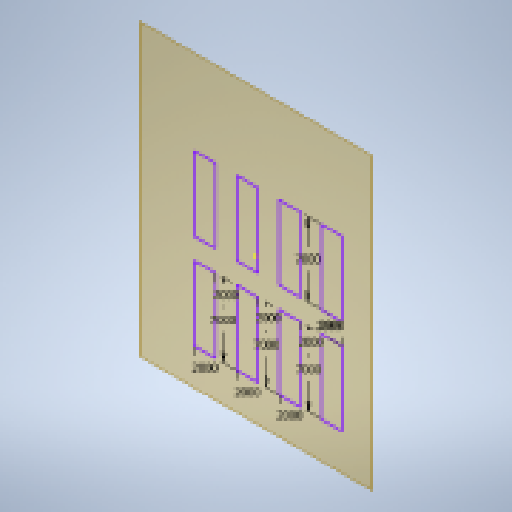
# Autodesk Inventor part: farm pot
Saved by Autodesk Inventor 2025 (Build 290162010, 162A)
## iProperties
Created: 2024-06-18
Part Number: farm pot
Material: 일반
Document SubType Name: Modeling
Designer: user
Density: 1 g/cm^3
Appearance: 기본값
Author: user
Autodesk Inventor part; units mm, degrees
ref_plane "YZ Plane" through (0, 0, 0) normal (1, 0, 0) x (0, 1, 0)
ref_plane "XZ Plane" through (0, 0, 0) normal (0, 1, 0) x (-1, 0, 0)
ref_plane "XY Plane" through (0, 0, 0) normal (0, 0, 1) x (1, 0, 0)
ref_plane "작업 평면1" through (0, 0, 0) normal (0, 0, 1) x (1, 0, 0)
ref_plane "작업 평면2" through (0, 0, 0) normal (0, 0, 1) x (1, 0, 0)
sketch "스케치1" plane through (0, 0, 0) normal (0, 0, 1) x (1, 0, 0)
  line L0 (8181.2099, -11309.2966) -> (6181.2099, -11309.2966)
  line L1 (6181.2099, -11309.2966) -> (6181.2099, -4309.2966)
  line L2 (6181.2099, -4309.2966) -> (8181.2099, -4309.2966)
  line L3 (8181.2099, -4309.2966) -> (8181.2099, -11309.2966)
  line L4 (4181.2099, -4309.2966) -> (2181.2099, -4309.2966)
  line L5 (2181.2099, -4309.2966) -> (2181.2099, -11309.2966)
  line L6 (2181.2099, -11309.2966) -> (4181.2099, -11309.2966)
  line L7 (4181.2099, -11309.2966) -> (4181.2099, -4309.2966)
  line L8 (181.2099, -4309.2966) -> (-1818.7901, -4309.2966)
  line L9 (-1818.7901, -4309.2966) -> (-1818.7901, -11309.2966)
  line L10 (-1818.7901, -11309.2966) -> (181.2099, -11309.2966)
  line L11 (181.2099, -11309.2966) -> (181.2099, -4309.2966)
  line L12 (-3818.7901, -4309.2966) -> (-5818.7901, -4309.2966)
  line L13 (-5818.7901, -4309.2966) -> (-5818.7901, -11309.2966)
  line L14 (-5818.7901, -11309.2966) -> (-3818.7901, -11309.2966)
  line L15 (-3818.7901, -11309.2966) -> (-3818.7901, -4309.2966)
  line L16 (8181.2099, -1299.5736) -> (6181.2099, -1299.5736)
  line L17 (6181.2099, -1299.5736) -> (6181.2099, 5700.4264)
  line L18 (6181.2099, 5700.4264) -> (8181.2099, 5700.4264)
  line L19 (8181.2099, 5700.4264) -> (8181.2099, -1299.5736)
  line L20 (4181.2099, -1299.5736) -> (2181.2099, -1299.5736)
  line L21 (2181.2099, -1299.5736) -> (2181.2099, 5700.4264)
  line L22 (2181.2099, 5700.4264) -> (4181.2099, 5700.4264)
  line L23 (4181.2099, 5700.4264) -> (4181.2099, -1299.5736)
  line L24 (181.2099, -1299.5736) -> (-1818.7901, -1299.5736)
  line L25 (-1818.7901, -1299.5736) -> (-1818.7901, 5700.4264)
  line L26 (-1818.7901, 5700.4264) -> (181.2099, 5700.4264)
  line L27 (181.2099, 5700.4264) -> (181.2099, -1299.5736)
  line L28 (-3818.7901, -1299.5741) -> (-5818.7901, -1299.5741)
  line L29 (-5818.7901, -1299.5741) -> (-5818.7901, 5700.4259)
  line L30 (-5818.7901, 5700.4259) -> (-3818.7901, 5700.4259)
  line L31 (-3818.7901, 5700.4259) -> (-3818.7901, -1299.5741)
  line L32 (8181.2099, -14311.8596) -> (6181.2099, -14311.8596)
  line L33 (6181.2099, -14311.8596) -> (6181.2099, -21311.8596)
  line L34 (6181.2099, -21311.8596) -> (8181.2099, -21311.8596)
  line L35 (8181.2099, -21311.8596) -> (8181.2099, -14311.8596)
  line L36 (4181.2099, -14311.8597) -> (2181.2099, -14311.8597)
  line L37 (2181.2099, -14311.8597) -> (2181.2099, -21311.8597)
  line L38 (2181.2099, -21311.8597) -> (4181.2099, -21311.8597)
  line L39 (4181.2099, -21311.8597) -> (4181.2099, -14311.8597)
  line L40 (181.2099, -14311.8597) -> (-1818.7901, -14311.8597)
  line L41 (-1818.7901, -14311.8597) -> (-1818.7901, -21311.8597)
  line L42 (-1818.7901, -21311.8597) -> (181.2099, -21311.8597)
  line L43 (181.2099, -21311.8597) -> (181.2099, -14311.8597)
  line L44 (-3818.7901, -14311.8597) -> (-5818.7901, -14311.8597)
  line L45 (-5818.7901, -14311.8597) -> (-5818.7901, -21311.8597)
  line L46 (-5818.7901, -21311.8597) -> (-3818.7901, -21311.8597)
  line L47 (-3818.7901, -21311.8597) -> (-3818.7901, -14311.8597)
  point P0 (0, 0)
  dimension "d0" = 2000
  dimension "d1" = 7000
  dimension "d2" = 2000
  dimension "d3" = 2000
  dimension "d4" = 7000
  dimension "d5" = 2000
  dimension "d6" = 2000
  dimension "d7" = 7000
  dimension "d8" = 2000
  dimension "d9" = 2000
  dimension "d10" = 3009.723
  dimension "d11" = 7000
  dimension "d12" = 3002.563
  dimension "d13" = 7000
  constraints: 96 end point, 24 parallel, 12 horizontal, 12 perpendicular, 8 point on line
  measures "d0" distance of L1.end L2.end
  measures "d1" distance of L0.end L1.end
  measures "d2" distance of L1.end L4.start
  measures "d3" distance of L6.end L5.end
  measures "d4" distance of L5.end L4.end
  measures "d5" distance of L4.end L8.start
  measures "d6" distance of L10.end L9.end
  measures "d7" distance of L9.end L8.end
  measures "d8" distance of L8.end L12.start
  measures "d9" distance of L14.end L13.end
  measures "d10" distance of L2.end L16.start
  measures "d11" distance of L16.end L17.end
  measures "d12" distance of L0.start L32.start
  measures "d13" distance of L33.end L32.end
extrude "돌출1" add sketch "스케치1" along normal blind 450
fillet "모깎기1" radius 50 48 edges at (-5818.7901, -1299.5741, 225) (-3818.7901, -1299.5741, 225) (-1818.7901, -1299.5736, 225) (181.2099, -1299.5736, 225) (2181.2099, -1299.5736, 225) (4181.2099, -1299.5736, 225) (6181.2099, -1299.5736, 225) (8181.2099, -1299.5736, 225) (-5818.7901, -11309.2966, 225) (-3818.7901, -11309.2966, 225) (-1818.7901, -11309.2966, 225) (181.2099, -11309.2966, 225) (2181.2099, -11309.2966, 225) (4181.2099, -11309.2966, 225) (6181.2099, -11309.2966, 225) (8181.2099, -11309.2966, 225) (-5818.7901, -21311.8597, 225) (-3818.7901, -21311.8597, 225) (-1818.7901, -21311.8597, 225) (181.2099, -21311.8597, 225) (2181.2099, -21311.8597, 225) (4181.2099, -21311.8597, 225) (6181.2099, -21311.8596, 225) (8181.2099, -21311.8596, 225) (8181.2099, -14311.8596, 225) (4181.2099, -14311.8597, 225) (6181.2099, -14311.8596, 225) (2181.2099, -14311.8597, 225) (181.2099, -14311.8597, 225) (-1818.7901, -14311.8597, 225) (-3818.7901, -14311.8597, 225) (-5818.7901, -14311.8597, 225) (-3818.7901, -4309.2966, 225) (-5818.7901, -4309.2966, 225) (181.2099, -4309.2966, 225) (-1818.7901, -4309.2966, 225) (-3818.7901, 5700.4259, 225) (-5818.7901, 5700.4259, 225) (181.2099, 5700.4264, 225) (-1818.7901, 5700.4264, 225) (4181.2099, 5700.4264, 225) (2181.2099, 5700.4264, 225) (4181.2099, -4309.2966, 225) (2181.2099, -4309.2966, 225) (8181.2099, -4309.2966, 225) (6181.2099, -4309.2966, 225) (8181.2099, 5700.4264, 225) (6181.2099, 5700.4264, 225)
sketch "스케치2" plane through (0, 0, 450) normal (0, 0, 1) x (1, 0, 0)
  arc A0 (4181.2099, 5650.4264) -> (4131.2099, 5700.4264) centre (4131.2099, 5650.4264) ccw projected
  arc A1 (2181.2099, -1249.5736) -> (2231.2099, -1299.5736) centre (2231.2099, -1249.5736) ccw projected
  line L0 (4131.2099, 5650.4264) -> (2231.2099, 5650.4264)
  line L1 (2231.2099, 5650.4264) -> (2231.2099, -1249.5736)
  line L2 (2231.2099, -1249.5736) -> (4131.2099, -1249.5736)
  line L3 (4131.2099, -1249.5736) -> (4131.2099, 5650.4264)
  arc A2 (8181.2099, 5650.4264) -> (8131.2099, 5700.4264) centre (8131.2099, 5650.4264) ccw projected
  line L4 (8131.2099, 5650.4264) -> (6231.2099, 5650.4264)
  line L5 (6231.2099, 5650.4264) -> (6231.2099, -1249.5736)
  line L6 (6231.2099, -1249.5736) -> (8131.2099, -1249.5736)
  line L7 (8131.2099, -1249.5736) -> (8131.2099, 5650.4264)
  arc A3 (6181.2099, -11259.2966) -> (6231.2099, -11309.2966) centre (6231.2099, -11259.2966) ccw projected
  line L8 (8131.2099, -4380.0511) -> (6231.2099, -4380.0511)
  line L9 (6231.2099, -4380.0511) -> (6231.2099, -11259.2966)
  line L10 (6231.2099, -11259.2966) -> (8131.2099, -11259.2966)
  line L11 (8131.2099, -11259.2966) -> (8131.2099, -4380.0511)
  arc A4 (8181.2099, -14361.8596) -> (8131.2099, -14311.8596) centre (8131.2099, -14361.8596) ccw projected
  arc A5 (6181.2099, -21261.8596) -> (6231.2099, -21311.8596) centre (6231.2099, -21261.8596) ccw projected
  line L12 (8131.2099, -14361.8596) -> (6231.2099, -14361.8596)
  line L13 (6231.2099, -14361.8596) -> (6231.2099, -21261.8596)
  line L14 (6231.2099, -21261.8596) -> (8131.2099, -21261.8596)
  line L15 (8131.2099, -21261.8596) -> (8131.2099, -14361.8596)
  arc A6 (4181.2099, -14361.8597) -> (4131.2099, -14311.8597) centre (4131.2099, -14361.8597) ccw projected
  arc A7 (2181.2099, -21261.8597) -> (2231.2099, -21311.8597) centre (2231.2099, -21261.8597) ccw projected
  line L16 (4131.2099, -14361.8597) -> (2231.2099, -14361.8597)
  line L17 (2231.2099, -14361.8597) -> (2231.2099, -21261.8597)
  line L18 (2231.2099, -21261.8597) -> (4131.2099, -21261.8597)
  line L19 (4131.2099, -21261.8597) -> (4131.2099, -14361.8597)
  arc A8 (4181.2099, -4359.2966) -> (4131.2099, -4309.2966) centre (4131.2099, -4359.2966) ccw projected
  arc A9 (2181.2099, -11259.2966) -> (2231.2099, -11309.2966) centre (2231.2099, -11259.2966) ccw projected
  line L20 (4131.2099, -4359.2966) -> (2231.2099, -4359.2966)
  line L21 (2231.2099, -4359.2966) -> (2231.2099, -11259.2966)
  line L22 (2231.2099, -11259.2966) -> (4131.2099, -11259.2966)
  line L23 (4131.2099, -11259.2966) -> (4131.2099, -4359.2966)
  arc A10 (181.2099, 5650.4264) -> (131.2099, 5700.4264) centre (131.2099, 5650.4264) ccw projected
  arc A11 (-1818.7901, -1249.5736) -> (-1768.7901, -1299.5736) centre (-1768.7901, -1249.5736) ccw projected
  line L24 (131.2099, 5650.4264) -> (-1768.7901, 5650.4264)
  line L25 (-1768.7901, 5650.4264) -> (-1768.7901, -1249.5736)
  line L26 (-1768.7901, -1249.5736) -> (131.2099, -1249.5736)
  line L27 (131.2099, -1249.5736) -> (131.2099, 5650.4264)
  arc A12 (181.2099, -4359.2966) -> (131.2099, -4309.2966) centre (131.2099, -4359.2966) ccw projected
  arc A13 (-1818.7901, -11259.2966) -> (-1768.7901, -11309.2966) centre (-1768.7901, -11259.2966) ccw projected
  line L28 (131.2099, -4359.2966) -> (-1768.7901, -4359.2966)
  line L29 (-1768.7901, -4359.2966) -> (-1768.7901, -11259.2966)
  line L30 (-1768.7901, -11259.2966) -> (131.2099, -11259.2966)
  line L31 (131.2099, -11259.2966) -> (131.2099, -4359.2966)
  arc A14 (181.2099, -14361.8597) -> (131.2099, -14311.8597) centre (131.2099, -14361.8597) ccw projected
  arc A15 (-1818.7901, -21261.8597) -> (-1768.7901, -21311.8597) centre (-1768.7901, -21261.8597) ccw projected
  line L32 (131.2099, -14361.8597) -> (-1768.7901, -14361.8597)
  line L33 (-1768.7901, -14361.8597) -> (-1768.7901, -21261.8597)
  line L34 (-1768.7901, -21261.8597) -> (131.2099, -21261.8597)
  line L35 (131.2099, -21261.8597) -> (131.2099, -14361.8597)
  arc A16 (-3818.7901, 5650.4259) -> (-3868.7901, 5700.4259) centre (-3868.7901, 5650.4259) ccw projected
  arc A17 (-5818.7901, -1249.5741) -> (-5768.7901, -1299.5741) centre (-5768.7901, -1249.5741) ccw projected
  line L36 (-3868.7901, 5650.4259) -> (-5768.7901, 5650.4259)
  line L37 (-5768.7901, 5650.4259) -> (-5768.7901, -1249.5741)
  line L38 (-5768.7901, -1249.5741) -> (-3868.7901, -1249.5741)
  line L39 (-3868.7901, -1249.5741) -> (-3868.7901, 5650.4259)
  arc A18 (-3818.7901, -4359.2966) -> (-3868.7901, -4309.2966) centre (-3868.7901, -4359.2966) ccw projected
  arc A19 (-5818.7901, -11259.2966) -> (-5768.7901, -11309.2966) centre (-5768.7901, -11259.2966) ccw projected
  line L40 (-3868.7901, -4359.2966) -> (-5768.7901, -4359.2966)
  line L41 (-5768.7901, -4359.2966) -> (-5768.7901, -11259.2966)
  line L42 (-5768.7901, -11259.2966) -> (-3868.7901, -11259.2966)
  line L43 (-3868.7901, -11259.2966) -> (-3868.7901, -4359.2966)
  arc A20 (-3818.7901, -14361.8597) -> (-3868.7901, -14311.8597) centre (-3868.7901, -14361.8597) ccw projected
  arc A21 (-5818.7901, -21261.8597) -> (-5768.7901, -21311.8597) centre (-5768.7901, -21261.8597) ccw projected
  line L44 (-3868.7901, -14361.8597) -> (-5768.7901, -14361.8597)
  line L45 (-5768.7901, -14361.8597) -> (-5768.7901, -21261.8597)
  line L46 (-5768.7901, -21261.8597) -> (-3868.7901, -21261.8597)
  line L47 (-3868.7901, -21261.8597) -> (-3868.7901, -14361.8597)
  point P0 (0, 0)
  constraints: 96 end point, 24 parallel, 12 horizontal, 12 perpendicular, 2 point on line
extrude "돌출2" cut sketch "스케치2" against normal blind 450
